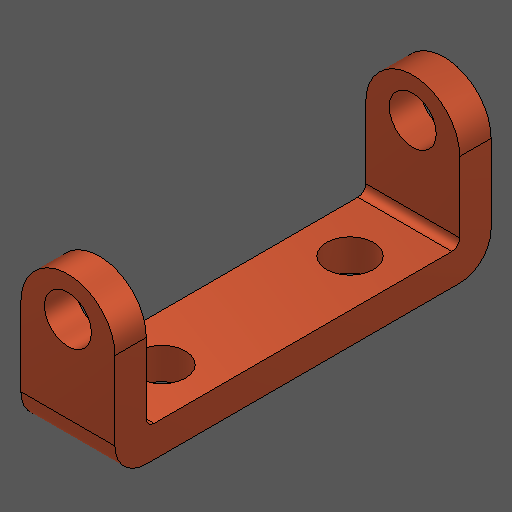
# Autodesk Inventor part: Plasma Box Hinge
Saved by Autodesk Inventor 2025 (Build 290162000, 162)
## iProperties
Created: 2023-12-08
Part Number: Plasma Box Hinge
Material: Generic
Document SubType Name: Modeling
Designer: jin20
Density: 1 g/cm^3
Appearance: 銅 - サテン
Author: jin20
Autodesk Inventor part; units mm, degrees
ref_plane "YZ Plane" through (0, 0, 0) normal (1, 0, 0) x (0, 1, 0)
ref_plane "XZ Plane" through (0, 0, 0) normal (0, 1, 0) x (-1, 0, 0)
ref_plane "XY Plane" through (0, 0, 0) normal (0, 0, 1) x (1, 0, 0)
sketch "スケッチ2" plane through (0, 0, 0) normal (0, 1, 0) x (-1, 0, 0)
  line L0 (3, 12) -> (-3, 12)
  line L1 (-3, 12) -> (-3, -12)
  line L2 (-3, -12) -> (3, -12)
  line L3 (3, -12) -> (3, 12)
  line L4 (3, 12) -> (-3, -12) construction
  line L5 (-3, 12) -> (3, -12) construction
  point P0 (0, 0)
  dimension "d0" = 6
  dimension "d1" = 24
  constraints: 12 end point, 2 midpoint, 2 parallel, 1 horizontal, 1 perpendicular
  measures "d0" distance of L2.end L1.end
  measures "d1" distance of L1.end L0.end
extrude "押し出し1" add sketch "スケッチ2" along normal blind 2
sketch "スケッチ3" plane through (0, 2, 0) normal (0, 1, 0) x (1, 0, 0)
  line L0 (0, 0) -> (17.0927, 0) construction
  circle A0 centre (0, -6) radius 1.5
  circle A1 centre (0, 6) radius 1.5
  dimension "d25" = 3
  constraints: 2 centre point, 2 end point, 1 horizontal, 1 symmetric about line, 1 other
  measures "d25" diameter of A0
extrude "押し出し2" cut sketch "スケッチ3" against normal through all
sketch "スケッチ4" plane through (0, 2, 0) normal (0, 1, 0) x (1, 0, 0)
  line L0 (-3, -12) -> (3, -12) projected
  line L1 (3, -12) -> (-3, -12)
  line L2 (-3, -12) -> (-3, -10)
  line L3 (-3, -10) -> (3, -10)
  line L4 (3, -10) -> (3, -12)
  line L5 (0, 0) -> (11.7228, 0) construction
  line L6 (-3, 12) -> (3, 12)
  line L7 (-3, 12) -> (-3, 10)
  line L8 (-3, 10) -> (3, 10)
  line L9 (3, 10) -> (3, 12)
  dimension "d8" = 6
  dimension "d9" = 2
  constraints: 18 end point, 5 symmetric about line, 2 horizontal, 2 parallel, 1 perpendicular
  measures "d8" distance of L2.end L3.end
  measures "d9" distance of L1.end L2.end
extrude "押し出し3" add sketch "スケッチ4" along normal blind 8
sketch "スケッチ6" plane through (-3, 0, 12) normal (0, 0, 1) x (1, 0, 0)
  circle A0 centre (3, 7.5) radius 1.5
  point P0 (3, 0)
  dimension "d36" = 3
  constraints: 1 centre point
  measures "d36" diameter of A0
extrude "押し出し4" cut sketch "スケッチ6" against normal through all
fillet "フィレット1" radius 2 1 edges at (0, 0, 12)
fillet "フィレット2" radius 0.5 1 edges at (0, 2, 10)
fillet "フィレット3" radius 0.5 1 edges at (0, 2, -10)
fillet "フィレット4" radius 2 1 edges at (0, 0, -12)
fillet "フィレット5" radius 3 4 edges at (3, 10, 11) (-3, 10, 11) (3, 10, -11) (-3, 10, -11)
